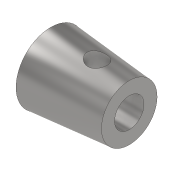
# Autodesk Inventor part: 旋塞
Saved by Autodesk Inventor 2022 (Build 260153000, 153)
## iProperties
Created: 2023-03-14
Part Number: 旋塞
Material: 不锈钢
Document SubType Name: Modeling
Designer: Lzy18
Density: 8 g/cm^3
Appearance: 半抛光
Author: Lzy18
Autodesk Inventor part; units mm, degrees
ref_plane "YZ Plane" through (0, 0, 0) normal (1, 0, 0) x (0, 1, 0)
ref_plane "XZ Plane" through (0, 0, 0) normal (0, 1, 0) x (-1, 0, 0)
ref_plane "XY Plane" through (0, 0, 0) normal (0, 0, 1) x (1, 0, 0)
sketch "草图1" plane through (0, 0, 0) normal (0, 0, 1) x (1, 0, 0)
  arc A0 (19, 0) -> (0, 35.6791) centre (-24, 0) ccw
  line L0 (96, 34) -> (96, 0)
  line L1 (96, 34) -> (0, 42.3989)
  line L2 (-101.2978, 0) -> (181.6605, 0)
  line L3 (0, 42.3989) -> (0, 35.6791)
  point P0 (0, 0)
  dimension "d0" = 24
  dimension "d1" = 86
  dimension "d2" = 34
  dimension "d4" = 5
  constraints: 8 end point, 2 horizontal, 2 point on circle, 2 point on line, 2 vertical, 1 centre point, 1 coincident
  measures "d0" distance of point (0, 0) point (-24, 0)
  measures "d1" diameter of A0
  measures "d2" distance of L0.end L0.start
  measures "d4" angle of L2 L1
revolve "旋转1" add sketch "草图1" angle 360 about axis through (-101.2978, 0, 0) along (1, 0, 0)
sketch "草图2" plane through (96, 0, 0) normal (1, 0, 0) x (0, 0, -1)
  circle A0 centre (0, 0) radius 34 projected
  point P0 (0, 0)
  constraints: 1 coincident
hole "孔1" at (96, 0, 0) direction (-1, 0, 0) diameter 36 depth 60
sketch "草图3" plane through (0, 0, 0) normal (0, 1, 0) x (-1, 0, 0)
  circle A0 centre (-56.72, 0) radius 12
  line L0 (-96, 34) -> (-96, -34) projected
  point P0 (0, 0)
  dimension "d13" = 24
  dimension "d14" = 39.28
  constraints: 1 centre point
  measures "d13" diameter of A0
  measures "d14" distance from line of L0 A0.centre
extrude "拉伸1" cut sketch "草图3" along normal up to surface
sketch "草图4" plane through (0, 0, 0) normal (0, 0, 1) x (1, 0, 0)
  line L0 (96, 18) -> (96, -18) projected
  line L1 (36, -18) -> (36, 18) projected
  circle A0 centre (57.0565, 0) radius 12
  point P0 (0, 0)
  point P1 (56.72, 13.4164)
  point P2 (56.72, 13.4164)
  point P3 (57.0565, 35.4317)
  dimension "d17" = 24
  constraints: 1 centre point
  measures "d17" diameter of A0
extrude "拉伸2" cut sketch "草图4" against normal up to surface
